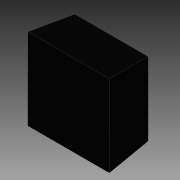
# Autodesk Inventor part: EPL2010-332ML
Saved by Autodesk Inventor 2013 (Build 170138000, 138)
## iProperties
Created: 2015-07-08
Part Number: EPL2010-332ML
Material: Ogólny
Document SubType Name: Modeling
Designer: terg
Density: 1 g/cm^3
Author: terg
Autodesk Inventor part; units mm, degrees
ref_plane "YZ Plane" through (0, 0, 0) normal (1, 0, 0) x (0, 1, 0)
ref_plane "XZ Plane" through (0, 0, 0) normal (0, 1, 0) x (-1, 0, 0)
ref_plane "XY Plane" through (0, 0, 0) normal (0, 0, 1) x (1, 0, 0)
sketch "Szkic1" plane through (0, 0, 0) normal (0, 1, 0) x (-1, 0, 0)
  line L0 (0, 0) -> (2, 0)
  line L1 (2, 0) -> (2, 2)
  line L2 (2, 2) -> (0, 2)
  line L3 (0, 2) -> (0, 0)
  dimension "d0" = 2
  dimension "d1" = 2
  constraints: 8 end point, 2 parallel, 1 horizontal, 1 perpendicular
  measures "d0" distance of L2.end L1.end
  measures "d1" distance of L1.end L0.end
extrude "Wyciągnięcie proste1" add sketch "Szkic1" along normal blind 1.05
chamfer "Faza1" distance 0.1 distance2 1.05 1 edges at (-1, 1.05, 2) measured on face at (-0.6667, 1.05, 1.3333)
chamfer "Faza2" distance 1.05 distance2 0.1 1 edges at (0, 1.05, 0.9503) measured on face at (0, 0.3502, 1.3002)
chamfer "Faza3" distance 1.05 distance2 0.1 1 edges at (-1.0497, 1.05, 0) measured on face at (-0.6998, 0.3502, 0)
chamfer "Faza4" distance 1.05 distance2 0.1 1 edges at (-2, 1.05, 1) measured on face at (-2, 0.3503, 0.6998)
sketch "Szkic2" plane through (0, 1.05, 0) normal (0, 1, 0) x (1, 0, 0)
  line L0 (-1.9, -1.9) -> (-1.9, -0.1) projected
  line L1 (-0.1, -1.9) -> (-1.9, -1.9) projected
  line L2 (-0.1, -0.1) -> (-0.1, -1.9) projected
  line L3 (-1.9, -0.1) -> (-0.1, -0.1) projected
  circle A0 centre (-1.45, -1) radius 0.1
  circle A1 centre (-0.55, -0.55) radius 0.1
  circle A2 centre (-0.55, -1.45) radius 0.1
  point P0 (0, 0)
  dimension "d16" = 0.45
  dimension "d17" = 1.8
  dimension "d18" = 0.9
  dimension "d19" = 0.45
  dimension "d20" = 0.45
  dimension "d21" = 0.45
  dimension "d22" = 0.45
  dimension "d23" = 0.2
  dimension "d24" = 0.2
  dimension "d25" = 0.2
  constraints: 3 centre point, 3 coincident
  measures "d16" distance from line of L0 point (-1.45, -1)
  measures "d17" distance of L0.end L2.start
  measures "d18" distance from line of L3 point (-1.45, -1)
  measures "d19" distance from line of L2 point (-0.55, -0.55)
  measures "d20" distance from line of L2 point (-0.55, -1.45)
  measures "d21" distance from line of L1 point (-0.55, -1.45)
  measures "d22" distance from line of L3 point (-0.55, -0.55)
  measures "d23" diameter of A0
  measures "d24" diameter of A1
  measures "d25" diameter of A2
extrude "Wyciągnięcie proste2" cut sketch "Szkic2" against normal blind 0.1 contours A0 | A1 | A2
equation "\"d16\" = 0.25 * d17"
equation "\"d18\" = 0.5 * d17"
equation "\"d19\" = d16"
equation "\"d20\" = d19"
equation "\"d21\" = d20"
equation "\"d22\" = d21"
